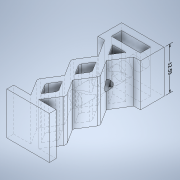
# Autodesk Inventor part: resorte2
Saved by Autodesk Inventor 2021.5 (Build 255421000, 421)
## iProperties
Created: 2024-11-28
Part Number: resorte2
Material: Genérico
Document SubType Name: Modeling
Designer: Joho_
Density: 1 g/cm^3
Appearance: Valor por defecto
Author: Joho_
## iProperties of the stored document _3DPrint.ipt
Created: 2024-11-28
Part Number: _3DPrint
Material: Genérico
Document SubType Name: Modeling
Designer: Joho_
Density: 1 g/cm^3
Appearance: Valor por defecto
Author: Joho_
Autodesk Inventor part; units mm, degrees
ref_plane "YZ Plane" through (0, 0, 0) normal (1, 0, 0) x (0, 1, 0)
ref_plane "XZ Plane" through (0, 0, 0) normal (0, 1, 0) x (-1, 0, 0)
ref_plane "XY Plane" through (0, 0, 0) normal (0, 0, 1) x (1, 0, 0)
sketch "Boceto1" plane through (0, 0, 0) normal (0, 0, 1) x (1, 0, 0)
  circle A0 centre (0, 0) radius 8.9
  line L0 (6.2933, -6.2933) -> (-6.2933, -6.2933)
  line L1 (-6.2933, -6.2933) -> (-6.2933, 6.2933)
  line L2 (-6.2933, 6.2933) -> (6.2933, 6.2933)
  line L3 (6.2933, 6.2933) -> (6.2933, -6.2933)
  dimension "d0" = 17.8
  dimension "d1" = 12.5865
  dimension "d2" = 12.5865
  constraints: 8 end point, 2 parallel, 1 centre point, 1 coincident, 1 horizontal, 1 perpendicular
  measures "d0" diameter of A0
  measures "d1" distance of L1.end L2.end
  measures "d2" distance of L0.end L1.end
extrude "Extrusión1" add sketch "Boceto1" along normal blind 32 contours L3 L0 L1 L2
sketch "Boceto3" plane through (0, 0, 0) normal (0, 0, -1) x (-1, 0, 0)
  circle A0 centre (0, 0) radius 2
  dimension "d25" = 4
  constraints: 1 centre point, 1 coincident
  measures "d25" diameter of A0
extrude "Extrusión3" cut sketch "Boceto3" against normal blind 20
sketch "Boceto4" plane through (0, 0, 0) normal (0, 1, 0) x (-1, 0, 0)
  line L0 (-6.2933, 0) -> (6.2933, 0) projected
  line L1 (-6.2933, 0) -> (6.2933, 0)
  line L2 (6.2933, 0) -> (6.2933, 2)
  line L3 (6.2933, 2) -> (-6.2933, 2)
  line L4 (-6.2933, 2) -> (-6.2933, 0)
  line L5 (-6.2933, 0) -> (-4.2933, 0)
  line L6 (-4.2933, 0) -> (-4.2933, 5)
  line L7 (-4.2933, 5) -> (-6.2933, 5)
  line L8 (-6.2933, 5) -> (-6.2933, 0)
  line L9 (6.2933, 0) -> (4.2933, 0)
  line L10 (4.2933, 0) -> (4.2933, 5)
  line L11 (4.2933, 5) -> (6.2933, 5)
  line L12 (6.2933, 5) -> (6.2933, 0)
  line L13 (-6.2933, 5) -> (6.2933, 5)
  line L14 (6.2933, 5) -> (6.2933, 7)
  line L15 (6.2933, 7) -> (-6.2933, 7)
  line L16 (-6.2933, 7) -> (-6.2933, 5)
  line L17 (0, 7) -> (6.2933, 7)
  line L18 (0, 7) -> (-6.2933, 7)
  line L19 (3.1484, 5.1198) -> (-3.993, 16.4674)
  line L20 (-4.8411, 17.815) -> (-3.9947, 18.3476)
  line L21 (4.8411, 6.185) -> (3.1484, 5.1198)
  line L22 (-5.1073, 15.7625) -> (-3.4147, 14.697)
  line L23 (3.9942, 27.532) -> (-0.0773, 34)
  line L24 (-3.4155, 39.303) -> (-5.1081, 38.2376)
  line L25 (-6.2933, 32) -> (6.2933, 32) projected
  line L26 (-6.2933, 32) -> (6.2933, 32)
  line L27 (6.2933, 32) -> (6.2933, 34)
  line L28 (6.2933, 34) -> (-6.2933, 34)
  line L29 (-6.2933, 34) -> (-6.2933, 32)
  line L30 (-1.6298, 16.4672) -> (4.8411, 6.185)
  line L31 (-1.6297, 17.5326) -> (3.9942, 26.4665)
  line L32 (-2.4406, 34) -> (1.6309, 27.532)
  line L33 (-2.4406, 34) -> (-0.0773, 34)
  line L34 (1.6309, 26.4665) -> (-3.9929, 17.5327)
  line L35 (0, 0) -> (0, -2)
  arc A0 (-1.6297, 17.5326) -> (-1.6298, 16.4672) centre (-0.7834, 16.9999) ccw
  arc A1 (-3.9929, 17.5327) -> (-3.993, 16.4674) centre (-3.1466, 17) ccw
  arc A2 (1.6309, 26.4665) -> (1.6309, 27.532) centre (0.7846, 26.9993) ccw
  arc A3 (3.9942, 26.4665) -> (3.9942, 27.532) centre (3.1479, 26.9993) ccw
  line L36 (-3.1484, 5.1198) -> (3.993, 16.4674)
  line L37 (-4.8411, 6.185) -> (-3.1484, 5.1198)
  line L38 (-3.9942, 27.532) -> (0.0773, 34)
  line L39 (1.6298, 16.4672) -> (-4.8411, 6.185)
  line L40 (1.6297, 17.5326) -> (-3.9942, 26.4665)
  line L41 (2.4406, 34) -> (-1.6309, 27.532)
  line L42 (2.4406, 34) -> (0.0773, 34)
  line L43 (-1.6309, 26.4665) -> (3.9929, 17.5327)
  arc A4 (1.6298, 16.4672) -> (1.6297, 17.5326) centre (0.7834, 16.9999) ccw
  arc A5 (3.993, 16.4674) -> (3.9929, 17.5327) centre (3.1466, 17) ccw
  arc A6 (-1.6309, 27.532) -> (-1.6309, 26.4665) centre (-0.7846, 26.9993) ccw
  arc A7 (-3.9942, 27.532) -> (-3.9942, 26.4665) centre (-3.1479, 26.9993) ccw
  point P0 (3.1466, 7)
  point P1 (-3.1466, 7)
  point P2 (0.0009, 22)
  point P3 (0, 32)
  point P4 (3.4147, 14.697)
  point P5 (-0.0009, 22)
  point P6 (3.9947, 18.3476)
  point P7 (-4.2933, 2)
  point P8 (4.2933, 2)
  point P9 (0, 10.1225)
  point P10 (1.9651, 7)
  point P11 (-1.9651, 7)
  point P12 (0, 13.8775)
  point P13 (0, 20.1215)
  point P14 (0, 30.1229)
  point P15 (0, 23.8757)
  point P16 (4.3282, 7)
  point P17 (1.1815, 12)
  point P18 (1.1816, 21.9986)
  point P19 (1.1816, 32)
  point P20 (-1.1816, 32)
  point P21 (-1.1816, 21.9986)
  point P22 (-1.1815, 12)
  point P23 (-4.3282, 7)
  dimension "d28" = 2
  dimension "d29" = 2
  dimension "d30" = 5
  dimension "d31" = 2
  dimension "d32" = 5
  dimension "d33" = 2
  dimension "d36" = 15
  dimension "d44" = 2
  dimension "d45" = 2
  dimension "d46" = 1
  constraints: 84 end point, 19 symmetric about line, 16 point on circle, 14 parallel, 8 centre point, 8 tangent, 7 perpendicular, 5 horizontal, 4 midpoint, 3 equal radius, 2 collinear, 2 point on line, 1 vertical, 4 other
  measures "d28" distance of L2.end L1.end
  measures "d29" distance of L7.end L6.end
  measures "d30" distance of L6.end L5.end
  measures "d31" distance of L10.end L11.end
  measures "d32" distance of L9.end L10.end
  measures "d33" distance of L14.end L13.end
  measures "d36" distance of L19.start L20.start
  measures "d44" distance of L24.end L24.start
  measures "d45" distance of L27.end L26.end
  measures "d46" radius of A0
extrude "Extrusión4" cut sketch "Boceto4" against normal mid plane 100 contours L4 L3 L6 L0 | L6 L3 L10 L0 | L8 L7 L6 L3 | L16 L15 L39 L37 L36 L19 L21 L30 L14 L11 L13 L7 | L10 L3 L2 L0 | L10 L11 L12 L3 | L39 L19 L36 L15 | L15 L36 L37 L39 | L39 L30 L36 L19 | L19 A1 L34 L40 L31 A0 L30 L39 | L36 L30 L15 L19 | L39 A4 L40 L31 L43 A5 L36 L30 | L30 L21 L19 L15 | L40 A7 L38 L32 L41 A6 L43 L34 | L34 L43 L31 L40 | L34 A2 L32 L41 L23 A3 L31 L43 | L38 L23 L25 | L25 L29 L28 L32 | L25 L41 L32 | L32 L28 L23 L38 | L41 L28 L27 L25 | L23 L38 L28 L41 | L23 L28 L38 keep common part
extrude "Extrusión5" add sketch "Boceto4" along normal mid plane 12.5865 contours L38 L23 L25 | L25 L29 L28 L32 | L32 L28 L23 L38 | L41 L28 L27 L25 | L23 L38 L28 L41 | L23 L28 L38
